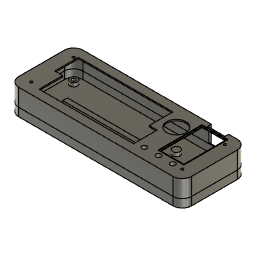
Macropad_V1_Case (Autodesk Fusion 360 design; units mm, degrees)
Autodesk Fusion 360 part; units mm, degrees
sketch "PCB" plane through (0, 0, 0) normal (0, 0, 1) x (1, 0, 0)
  line L0 (0, 0) -> (129.54, 0)
  line L1 (129.54, 0) -> (129.54, 41.91)
  line L2 (129.54, 41.91) -> (0, 41.91)
  line L3 (0, 41.91) -> (0, 0)
  circle A0 centre (3.81, 38.1) radius 1
  circle A1 centre (3.81, 3.81) radius 1
  circle A2 centre (125.73, 3.81) radius 1
  circle A3 centre (125.73, 38.1) radius 1
  line L4 (7.62, 38.1) -> (22.86, 38.1)
  line L5 (22.86, 38.1) -> (22.86, 22.86)
  line L6 (22.86, 22.86) -> (7.62, 22.86)
  line L7 (7.62, 22.86) -> (7.62, 38.1)
  line L8 (26.67, 22.86) -> (26.67, 38.1)
  line L9 (26.67, 38.1) -> (41.91, 38.1)
  line L10 (41.91, 38.1) -> (41.91, 22.86)
  line L11 (41.91, 22.86) -> (26.67, 22.86)
  line L12 (45.72, 22.86) -> (45.72, 38.1)
  line L13 (45.72, 38.1) -> (60.96, 38.1)
  line L14 (60.96, 38.1) -> (60.96, 22.86)
  line L15 (60.96, 22.86) -> (45.72, 22.86)
  line L16 (64.77, 22.86) -> (64.77, 38.1)
  line L17 (64.77, 38.1) -> (80.01, 38.1)
  line L18 (80.01, 38.1) -> (80.01, 22.86)
  line L19 (80.01, 22.86) -> (64.77, 22.86)
  line L20 (13.97, 19.05) -> (29.21, 19.05)
  line L21 (29.21, 19.05) -> (29.21, 3.81)
  line L22 (29.21, 3.81) -> (13.97, 3.81)
  line L23 (13.97, 3.81) -> (13.97, 19.05)
  line L24 (33.02, 3.81) -> (33.02, 19.05)
  line L25 (33.02, 19.05) -> (48.26, 19.05)
  line L26 (48.26, 19.05) -> (48.26, 3.81)
  line L27 (48.26, 3.81) -> (33.02, 3.81)
  line L28 (52.07, 3.81) -> (52.07, 19.05)
  line L29 (52.07, 19.05) -> (67.31, 19.05)
  line L30 (67.31, 19.05) -> (67.31, 3.81)
  line L31 (67.31, 3.81) -> (52.07, 3.81)
  line L32 (71.12, 3.81) -> (71.12, 19.05)
  line L33 (71.12, 19.05) -> (86.36, 19.05)
  line L34 (86.36, 19.05) -> (86.36, 3.81)
  line L35 (86.36, 3.81) -> (71.12, 3.81)
  line L36 (104.14, 41.91) -> (121.92, 41.91)
  line L37 (121.92, 41.91) -> (121.92, 8.89)
  line L38 (121.92, 8.89) -> (104.14, 8.89)
  line L39 (104.14, 8.89) -> (104.14, 41.91)
  line L40 (115.65, 6.27) -> (120.65, 6.27)
  line L41 (120.65, 6.27) -> (120.65, 1.27)
  line L42 (120.65, 1.27) -> (115.65, 1.27)
  line L43 (115.65, 1.27) -> (115.65, 6.27)
  line L44 (104.22, 1.27) -> (104.22, 6.27)
  line L45 (104.22, 6.27) -> (109.22, 6.27)
  line L46 (109.22, 6.27) -> (109.22, 1.27)
  line L47 (109.22, 1.27) -> (104.22, 1.27)
  line L48 (92.79, 1.27) -> (92.79, 6.27)
  line L49 (92.79, 6.27) -> (97.79, 6.27)
  line L50 (97.79, 6.27) -> (97.79, 1.27)
  line L51 (97.79, 1.27) -> (92.79, 1.27)
  circle A4 centre (93.98, 30.734) radius 3.81
  dimension "d1" = 129.54
  dimension "d2" = 41.91
  dimension "d38" = 2
  dimension "d39" = 3.81
  dimension "d40" = 3.81
  dimension "d41" = 2
  dimension "d42" = 3.81
  dimension "d43" = 3.81
  dimension "d44" = 2
  dimension "d45" = 3.81
  dimension "d46" = 3.81
  dimension "d47" = 2
  dimension "d48" = 3.81
  dimension "d49" = 3.81
  dimension "d50" = 15.24
  dimension "d51" = 15.24
  dimension "d52" = 7.62
  dimension "d53" = 3.81
  dimension "d56" = 19.05
  dimension "d57" = 0
  dimension "d58" = 15.24
  dimension "d59" = 15.24
  dimension "d60" = 19.05
  dimension "d61" = 6.35
  dimension "d64" = 19.05
  dimension "d65" = 0
  dimension "d66" = 17.78
  dimension "d67" = 33.02
  dimension "d68" = 7.62
  dimension "d71" = 5
  dimension "d72" = 5
  dimension "d73" = 8.89
  dimension "d74" = 1.27
  dimension "d77" = -11.43
  dimension "d78" = 0
  dimension "d79" = 7.62
  dimension "d80" = 35.56
  dimension "d81" = 11.176
  constraint horizontal L0
  constraint vertical L1
  constraint horizontal L2
  constraint vertical L3
  constraint coincident L0.start L3.end
  constraint horizontal L4
  constraint vertical L5
  constraint horizontal L6
  constraint vertical L7
  constraint horizontal L20
  constraint vertical L21
  constraint horizontal L22
  constraint vertical L23
  constraint horizontal L36
  constraint vertical L37
  constraint horizontal L38
  constraint vertical L39
  constraint collinear L2 L36
  constraint horizontal L40
  constraint vertical L41
  constraint horizontal L42
  constraint vertical L43
  measures "d1" distance of L0.start L0.end
  measures "d2" distance of L0.start L2.end
  measures "d38" diameter of A0
  measures "d39" distance of L3 A0.centre
  measures "d40" distance of L2 A0.centre
  measures "d41" diameter of A1
  measures "d42" distance of L0 A1.centre
  measures "d43" distance of L3 A1.centre
  measures "d44" diameter of A2
  measures "d45" distance of L1 A2.centre
  measures "d46" distance of L0 A2.centre
  measures "d47" diameter of A3
  measures "d48" distance of L2 A3.centre
  measures "d49" distance of L1 A3.centre
  measures "d50" distance of L4.start L4.end
  measures "d51" distance of L4.start L6.end
  measures "d52" distance of L3 L7
  measures "d53" distance of L2 L4
  measures "d58" distance of L20.end L20.start
  measures "d59" distance of L22.end L20.start
  measures "d60" distance of L4 L20
  measures "d61" distance of L7 L23
  measures "d66" distance of L36.start L36.end
  measures "d67" distance of L36.start L38.end
  measures "d68" distance of L1 L37
  measures "d71" distance of L40.start L40.end
  measures "d72" distance of L40.start L42.end
  measures "d73" distance of L1 L41
  measures "d74" distance of L0 L42
  measures "d79" diameter of A4
  measures "d80" distance of L1 A4.centre
  measures "d81" distance of L2 A4.centre
sketch "Bottom" plane through (0, 0, 0) normal (0, 0, 1) x (1, 0, 0)
  line L0 (2.5, 46.91) -> (127.04, 46.91)
  line L1 (134.54, 39.41) -> (134.54, 2.5)
  line L2 (127.04, -5) -> (2.5, -5)
  line L3 (-5, 2.5) -> (-5, 39.41)
  line L4 (0, 41.91) -> (0, 0)
  line L5 (129.54, 0) -> (129.54, 41.91)
  line L6 (129.54, 41.91) -> (0, 41.91)
  line L7 (0, 0) -> (129.54, 0)
  arc A0 (2.5, 46.91) -> (-5, 39.41) centre (2.5, 39.41) ccw
  arc A1 (134.54, 39.41) -> (127.04, 46.91) centre (127.04, 39.41) ccw
  arc A2 (127.04, -5) -> (134.54, 2.5) centre (127.04, 2.5) ccw
  arc A3 (-5, 2.5) -> (2.5, -5) centre (2.5, 2.5) ccw
  dimension "d9" = 5
  dimension "d10" = 5
  dimension "d11" = 5
  dimension "d12" = 5
  dimension "d13" = 7.5
  constraint horizontal L0
  constraint vertical L1
  constraint horizontal L2
  constraint vertical L3
  constraint tangent L3 A0
  constraint tangent L0 A0
  constraint tangent L0 A1
  constraint tangent L1 A1
  constraint equal A0 A1
  constraint tangent L1 A2
  constraint tangent L2 A2
  constraint equal A0 A2
  constraint tangent L2 A3
  constraint tangent L3 A3
  constraint equal A0 A3
  measures "d9" distance of L3 L4
  measures "d10" distance of L1 L5
  measures "d11" distance of L0 L6
  measures "d12" distance of L2 L7
  measures "d13" radius of A0
extrude "Extrude1" add sketch "Bottom" along normal blind 6.6 contours L0 L1 L2 L3 A0 A1 A2 A3 | L4 L5 L6 L7 makes body 1
sketch "Bottom indent" plane through (0, 0, 6.6) normal (0, 0, 1) x (-1, 0, 0)
  arc A0 (-2.5, -46.91) -> (5, -39.41) centre (-2.5, -39.41) ccw
  line L0 (5, -39.41) -> (5, -2.5)
  arc A1 (5, -2.5) -> (-2.5, 5) centre (-2.5, -2.5) ccw
  line L1 (-2.5, 5) -> (-127.04, 5)
  arc A2 (-127.04, 5) -> (-134.54, -2.5) centre (-127.04, -2.5) ccw
  line L2 (-134.54, -2.5) -> (-134.54, -39.41)
  arc A3 (-134.54, -39.41) -> (-127.04, -46.91) centre (-127.04, -39.41) ccw
  line L3 (-127.04, -46.91) -> (-2.5, -46.91)
  line L4 (-4.5, -44.91) -> (-125.04, -44.91)
  line L5 (-132.54, -37.41) -> (-132.54, -4.5)
  line L6 (-125.04, 3) -> (-4.5, 3)
  line L7 (3, -4.5) -> (3, -37.41)
  arc A4 (-4.5, -44.91) -> (3, -37.41) centre (-4.5, -37.41) ccw
  arc A5 (-132.54, -37.41) -> (-125.04, -44.91) centre (-125.04, -37.41) ccw
  arc A6 (-125.04, 3) -> (-132.54, -4.5) centre (-125.04, -4.5) ccw
  arc A7 (3, -4.5) -> (-4.5, 3) centre (-4.5, -4.5) ccw
  dimension "d17" = 2
  dimension "d18" = 2
  dimension "d19" = 2
  dimension "d20" = 2
  dimension "d21" = 7.5
  constraint horizontal L4
  constraint vertical L5
  constraint horizontal L6
  constraint vertical L7
  constraint tangent L7 A4
  constraint tangent L4 A4
  constraint tangent L4 A5
  constraint tangent L5 A5
  constraint equal A4 A5
  constraint tangent L5 A6
  constraint tangent L6 A6
  constraint equal A4 A6
  constraint tangent L6 A7
  constraint tangent L7 A7
  constraint equal A4 A7
  measures "d17" distance of L0 L7
  measures "d18" distance of L2 L5
  measures "d19" distance of L3 L4
  measures "d20" distance of L1 L6
  measures "d21" radius of A4
extrude "Extrude2" cut sketch "Bottom indent" against normal blind 4.6 contours L4 L5 L6 L7 A4 A5 A6 A7 bodies 1
sketch "Feet holes" plane through (0, 0, 0) normal (0, 0, -1) x (1, 0, 0)
  arc A0 (-5, -39.41) -> (2.5, -46.91) centre (2.5, -39.41) ccw
  line L0 (2.5, -46.91) -> (127.04, -46.91)
  arc A1 (127.04, -46.91) -> (134.54, -39.41) centre (127.04, -39.41) ccw
  line L1 (134.54, -39.41) -> (134.54, -2.5)
  arc A2 (134.54, -2.5) -> (127.04, 5) centre (127.04, -2.5) ccw
  line L2 (127.04, 5) -> (2.5, 5)
  arc A3 (2.5, 5) -> (-5, -2.5) centre (2.5, -2.5) ccw
  line L3 (-5, -2.5) -> (-5, -39.41)
  circle A4 centre (5, -5) radius 5
  circle A5 centre (5, -36.91) radius 5
  circle A6 centre (124.54, -5) radius 5
  circle A7 centre (124.54, -36.91) radius 5
  dimension "d24" = 10
  dimension "d25" = 10
  dimension "d26" = 10
  dimension "d27" = 10
  dimension "d28" = 10
  dimension "d29" = 10
  dimension "d30" = 10
  dimension "d31" = 10
  dimension "d32" = 10
  dimension "d33" = 10
  dimension "d34" = 10
  dimension "d35" = 10
  measures "d24" diameter of A4
  measures "d25" distance of L2 A4.centre
  measures "d26" distance of L3 A4.centre
  measures "d27" diameter of A5
  measures "d28" diameter of A6
  measures "d29" diameter of A7
  measures "d30" distance of L3 A5.centre
  measures "d31" distance of L0 A5.centre
  measures "d32" distance of L1 A6.centre
  measures "d33" distance of L2 A6.centre
  measures "d34" distance of L1 A7.centre
  measures "d35" distance of L0 A7.centre
extrude "Extrude3" cut sketch "Feet holes" against normal blind 1 contours A4 | A5 | A6 | A7 bodies 1
sketch "Bottom risers" plane through (0, 0, 2) normal (0, 0, 1) x (-1, 0, 0)
  arc A0 (-4.5, -44.91) -> (3, -37.41) centre (-4.5, -37.41) ccw
  line L0 (3, -37.41) -> (3, -4.5)
  arc A1 (3, -4.5) -> (-4.5, 3) centre (-4.5, -4.5) ccw
  line L1 (-4.5, 3) -> (-125.04, 3)
  arc A2 (-125.04, 3) -> (-132.54, -4.5) centre (-125.04, -4.5) ccw
  line L2 (-132.54, -4.5) -> (-132.54, -37.41)
  arc A3 (-132.54, -37.41) -> (-125.04, -44.91) centre (-125.04, -37.41) ccw
  line L3 (-125.04, -44.91) -> (-4.5, -44.91)
  circle A4 centre (-3.81, -38.1) radius 3
  circle A5 centre (-3.81, -38.1) radius 1
  circle A6 centre (-3.81, -3.81) radius 3
  circle A7 centre (-125.73, -38.1) radius 3
  circle A8 centre (-125.73, -3.81) radius 3
  circle A9 centre (-3.81, -3.81) radius 1
  circle A10 centre (-125.73, -38.1) radius 1
  circle A11 centre (-125.73, -3.81) radius 1
  line L4 (-13.97, -22.86) -> (-80.01, -22.86)
  line L5 (-80.01, -22.86) -> (-80.01, -19.05)
  line L6 (-80.01, -19.05) -> (-13.97, -19.05)
  line L7 (-13.97, -19.05) -> (-13.97, -22.86)
  line L8 (-80.01, -38.1) -> (-80.01, -22.86)
  line L9 (-13.97, -3.81) -> (-13.97, -19.05)
  line L10 (-13.97, -19.05) -> (-29.21, -19.05)
  line L11 (-80.01, -22.86) -> (-64.77, -22.86)
  circle A12 centre (-93.98, -30.734) radius 3
  circle A13 centre (-93.98, -30.734) radius 3.81
  circle A14 centre (-3.81, -38.1) radius 1.5
  circle A15 centre (-3.81, -3.81) radius 1.5
  circle A16 centre (-125.73, -3.81) radius 1.5
  circle A17 centre (-125.73, -38.1) radius 1.5
  dimension "d82" = 6
  dimension "d83" = 6
  dimension "d84" = 6
  dimension "d85" = 6
  dimension "d87" = 6
  dimension "d88" = 3
  dimension "d89" = 3
  dimension "d90" = 3
  dimension "d91" = 3
  constraint concentric A4 A5
  constraint concentric A6 A9
  constraint concentric A7 A10
  constraint concentric A8 A11
  constraint horizontal L4
  constraint vertical L5
  constraint horizontal L6
  constraint vertical L7
  constraint collinear L5 L8
  constraint collinear L7 L9
  constraint collinear L6 L10
  constraint collinear L4 L11
  constraint concentric A12 A13
  constraint concentric A5 A14
  constraint concentric A9 A15
  constraint concentric A11 A16
  constraint concentric A10 A17
  measures "d82" diameter of A4
  measures "d83" diameter of A6
  measures "d84" diameter of A7
  measures "d85" diameter of A8
  measures "d87" diameter of A12
  measures "d88" diameter of A14
  measures "d89" diameter of A15
  measures "d90" diameter of A16
  measures "d91" diameter of A17
extrude "Extrude4" add sketch "Bottom risers" along normal blind 3 contours A4 | A6 | A7 | A8 | L4 L5 L6 L7 L10 L11 | A12 bodies 1
extrude "Extrude5" cut 4 faces at (4.4705, 37.7379, 2) (3.6858, 4.5903, 2) (125.6187, 38.5875, 2) (126.2643, 4.2009, 2) along direction (0, 0, -1) blind 1 on bodies 1 bodies 1
sketch "Bottom Raised Edge" plane through (0, 0, 6.6) normal (0, 0, 1) x (-1, 0, 0)
  line L0 (3, -4.5) -> (3, -37.41)
  arc A0 (-4.5, -44.91) -> (3, -37.41) centre (-4.5, -37.41) ccw
  line L1 (-4.5, -44.91) -> (-125.04, -44.91)
  arc A1 (-132.54, -37.41) -> (-125.04, -44.91) centre (-125.04, -37.41) ccw
  line L2 (-132.54, -37.41) -> (-132.54, -4.5)
  arc A2 (-125.04, 3) -> (-132.54, -4.5) centre (-125.04, -4.5) ccw
  line L3 (-125.04, 3) -> (-4.5, 3)
  arc A3 (3, -4.5) -> (-4.5, 3) centre (-4.5, -4.5) ccw
  arc A4 (-2.5, -46.91) -> (5, -39.41) centre (-2.5, -39.41) ccw
  line L4 (5, -39.41) -> (5, -2.5)
  arc A5 (5, -2.5) -> (-2.5, 5) centre (-2.5, -2.5) ccw
  line L5 (-2.5, 5) -> (-127.04, 5)
  arc A6 (-127.04, 5) -> (-134.54, -2.5) centre (-127.04, -2.5) ccw
  line L6 (-134.54, -2.5) -> (-134.54, -39.41)
  arc A7 (-134.54, -39.41) -> (-127.04, -46.91) centre (-127.04, -39.41) ccw
  line L7 (-127.04, -46.91) -> (-2.5, -46.91)
  line L8 (-3.7, -45.71) -> (-125.84, -45.71)
  line L9 (-133.34, -38.21) -> (-133.34, -3.7)
  line L10 (-125.84, 3.8) -> (-3.7, 3.8)
  line L11 (3.8, -3.7) -> (3.8, -38.21)
  arc A8 (-3.7, -45.71) -> (3.8, -38.21) centre (-3.7, -38.21) ccw
  arc A9 (-133.34, -38.21) -> (-125.84, -45.71) centre (-125.84, -38.21) ccw
  arc A10 (-125.84, 3.8) -> (-133.34, -3.7) centre (-125.84, -3.7) ccw
  arc A11 (3.8, -3.7) -> (-3.7, 3.8) centre (-3.7, -3.7) ccw
  dimension "d96" = 0.8
  dimension "d97" = 0.8
  dimension "d98" = 0.8
  dimension "d100" = 0.8
  dimension "d101" = 7.5
  constraint horizontal L8
  constraint vertical L9
  constraint horizontal L10
  constraint vertical L11
  constraint tangent L8 A8
  constraint tangent L11 A8
  constraint tangent L8 A9
  constraint tangent L9 A9
  constraint equal A8 A9
  constraint tangent L9 A10
  constraint tangent L10 A10
  constraint equal A8 A10
  constraint tangent L10 A11
  constraint tangent L11 A11
  constraint equal A8 A11
  measures "d96" distance of L1 L8
  measures "d97" distance of L0 L11
  measures "d98" distance of L2 L9
  measures "d100" distance of L3 L10
  measures "d101" radius of A8
extrude "Extrude6" add sketch "Bottom Raised Edge" along normal blind 1.4 contours L8 L9 L10 L11 A8 A9 A10 A11 bodies 1
sketch "Top" plane through (0, 0, 6.6) normal (0, 0, 1) x (-1, 0, 0)
  line L0 (-3.7, -45.71) -> (-125.84, -45.71)
  arc A0 (-133.34, -38.21) -> (-125.84, -45.71) centre (-125.84, -38.21) ccw
  line L1 (-133.34, -38.21) -> (-133.34, -3.7)
  arc A1 (-125.84, 3.8) -> (-133.34, -3.7) centre (-125.84, -3.7) ccw
  line L2 (-125.84, 3.8) -> (-3.7, 3.8)
  arc A2 (3.8, -3.7) -> (-3.7, 3.8) centre (-3.7, -3.7) ccw
  line L3 (3.8, -3.7) -> (3.8, -38.21)
  arc A3 (-3.7, -45.71) -> (3.8, -38.21) centre (-3.7, -38.21) ccw
  arc A4 (-2.5, -46.91) -> (5, -39.41) centre (-2.5, -39.41) ccw
  line L4 (5, -39.41) -> (5, -2.5)
  arc A5 (5, -2.5) -> (-2.5, 5) centre (-2.5, -2.5) ccw
  line L5 (-2.5, 5) -> (-127.04, 5)
  arc A6 (-127.04, 5) -> (-134.54, -2.5) centre (-127.04, -2.5) ccw
  line L6 (-134.54, -2.5) -> (-134.54, -39.41)
  arc A7 (-134.54, -39.41) -> (-127.04, -46.91) centre (-127.04, -39.41) ccw
  line L7 (-127.04, -46.91) -> (-2.5, -46.91)
  line L8 (-2.5, -46.91) -> (-127.04, -46.91)
  line L9 (-134.54, -39.41) -> (-134.54, -2.5)
  line L10 (-127.04, 5) -> (-2.5, 5)
  line L11 (5, -2.5) -> (5, -39.41)
  arc A8 (-2.5, -46.91) -> (5, -39.41) centre (-2.5, -39.41) ccw
  arc A9 (-134.54, -39.41) -> (-127.04, -46.91) centre (-127.04, -39.41) ccw
  arc A10 (-127.04, 5) -> (-134.54, -2.5) centre (-127.04, -2.5) ccw
  arc A11 (5, -2.5) -> (-2.5, 5) centre (-2.5, -2.5) ccw
  dimension "d105" = 7.5
  constraint horizontal L8
  constraint vertical L9
  constraint horizontal L10
  constraint vertical L11
  constraint collinear L7 L8
  constraint collinear L4 L11
  constraint collinear L5 L10
  constraint collinear L6 L9
  constraint tangent L8 A8
  constraint tangent L11 A8
  constraint tangent L8 A9
  constraint tangent L9 A9
  constraint equal A8 A9
  constraint tangent L9 A10
  constraint tangent L10 A10
  constraint equal A8 A10
  constraint tangent L10 A11
  constraint tangent L11 A11
  constraint equal A8 A11
  measures "d105" radius of A8
extrude "Extrude7" add sketch "Top" along normal blind 14 separate body contours L0 A0 L1 A1 L2 A2 L3 A3 | A4 L4 A5 L5 A6 L6 A7 L7 L8 L9 L10 L11 A8 A9 A10 A11 makes body 2
sketch "Top Indent" plane through (0, 0, 6.6) normal (0, 0, -1) x (1, 0, 0)
  arc A0 (-5, -39.41) -> (2.5, -46.91) centre (2.5, -39.41) ccw
  line L0 (2.5, -46.91) -> (127.04, -46.91)
  arc A1 (127.04, -46.91) -> (134.54, -39.41) centre (127.04, -39.41) ccw
  line L1 (134.54, -39.41) -> (134.54, -2.5)
  arc A2 (134.54, -2.5) -> (127.04, 5) centre (127.04, -2.5) ccw
  line L2 (127.04, 5) -> (2.5, 5)
  arc A3 (2.5, 5) -> (-5, -2.5) centre (2.5, -2.5) ccw
  line L3 (-5, -2.5) -> (-5, -39.41)
  line L4 (4.5, 3) -> (125.04, 3)
  line L5 (132.54, -4.5) -> (132.54, -37.41)
  line L6 (125.04, -44.91) -> (4.5, -44.91)
  line L7 (-3, -37.41) -> (-3, -4.5)
  arc A4 (4.5, 3) -> (-3, -4.5) centre (4.5, -4.5) ccw
  arc A5 (132.54, -4.5) -> (125.04, 3) centre (125.04, -4.5) ccw
  arc A6 (125.04, -44.91) -> (132.54, -37.41) centre (125.04, -37.41) ccw
  arc A7 (-3, -37.41) -> (4.5, -44.91) centre (4.5, -37.41) ccw
  dimension "d109" = 2
  dimension "d110" = 2
  dimension "d111" = 2
  dimension "d112" = 2
  dimension "d113" = 7.5
  constraint horizontal L4
  constraint vertical L5
  constraint horizontal L6
  constraint vertical L7
  constraint tangent L4 A4
  constraint tangent L7 A4
  constraint tangent L4 A5
  constraint tangent L5 A5
  constraint equal A4 A5
  constraint tangent L5 A6
  constraint tangent L6 A6
  constraint equal A4 A6
  constraint tangent L6 A7
  constraint tangent L7 A7
  constraint equal A4 A7
  measures "d109" distance of L2 L4
  measures "d110" distance of L0 L6
  measures "d111" distance of L3 L7
  measures "d112" distance of L1 L5
  measures "d113" radius of A4
extrude "Extrude8" cut sketch "Top Indent" against normal blind 13 contours L4 L5 L6 L7 A4 A5 A6 A7 bodies 2
sketch "Top Light Pipes" plane through (0, 0, 19.6) normal (0, 0, -1) x (1, 0, 0)
  arc A0 (4.5, 3) -> (-3, -4.5) centre (4.5, -4.5) ccw
  line L0 (-3, -4.5) -> (-3, -37.41)
  arc A1 (-3, -37.41) -> (4.5, -44.91) centre (4.5, -37.41) ccw
  line L1 (4.5, -44.91) -> (125.04, -44.91)
  arc A2 (125.04, -44.91) -> (132.54, -37.41) centre (125.04, -37.41) ccw
  line L2 (132.54, -37.41) -> (132.54, -4.5)
  arc A3 (132.54, -4.5) -> (125.04, 3) centre (125.04, -4.5) ccw
  line L3 (125.04, 3) -> (4.5, 3)
  circle A4 centre (118.15, -3.77) radius 3
  circle A5 centre (-95.29, -3.77) radius 2
  circle A6 centre (106.72, -3.77) radius 3
  circle A7 centre (95.29, -3.77) radius 3
  line L4 (115.65, -6.27) -> (120.65, -6.27)
  line L5 (115.65, -1.27) -> (115.65, -6.27)
  line L6 (104.22, -6.27) -> (109.22, -6.27)
  line L7 (104.22, -1.27) -> (104.22, -6.27)
  line L8 (92.79, -6.27) -> (97.79, -6.27)
  line L9 (92.79, -1.27) -> (92.79, -6.27)
  dimension "d168" = 6
  dimension "d169" = 4
  dimension "d170" = 6
  dimension "d171" = 6
  dimension "d172" = 2.5
  dimension "d173" = 2.5
  dimension "d174" = 2.5
  dimension "d175" = 2.5
  dimension "d176" = 2.5
  dimension "d177" = 2.5
  measures "d168" diameter of A4
  measures "d169" diameter of A5
  measures "d170" diameter of A6
  measures "d171" diameter of A7
  measures "d172" distance of A4.centre L4
  measures "d173" distance of A4.centre L5
  measures "d174" distance of A6.centre L6
  measures "d175" distance of A6.centre L7
  measures "d176" distance of A7.centre L8
  measures "d177" distance of A7.centre L9
extrude "Extrude12" add sketch "Top Light Pipes" along normal blind 11 contours A4 L4 L5 | A4 L5 | A4 L4 | A6 L6 L7 | A6 L7 | A6 L6 | A7 L8 L9 | A7 L9 | A7 L8 picked at (118.1589, -4.4367) picked at (106.7289, -4.4367) picked at (95.2989, -4.4367) bodies 2
sketch "Top Key Holes" plane through (0, 0, 20.6) normal (0, 0, 1) x (-1, 0, 0)
  arc A0 (-2.5, -46.91) -> (5, -39.41) centre (-2.5, -39.41) ccw
  line L0 (5, -39.41) -> (5, -2.5)
  arc A1 (5, -2.5) -> (-2.5, 5) centre (-2.5, -2.5) ccw
  line L1 (-2.5, 5) -> (-127.04, 5)
  arc A2 (-127.04, 5) -> (-134.54, -2.5) centre (-127.04, -2.5) ccw
  line L2 (-134.54, -2.5) -> (-134.54, -39.41)
  arc A3 (-134.54, -39.41) -> (-127.04, -46.91) centre (-127.04, -39.41) ccw
  line L3 (-127.04, -46.91) -> (-2.5, -46.91)
  line L4 (-5.715, -40.005) -> (-24.765, -40.005)
  line L5 (-24.765, -40.005) -> (-24.765, -20.955)
  line L6 (-24.765, -20.955) -> (-5.715, -20.955)
  line L7 (-5.715, -20.955) -> (-5.715, -40.005)
  line L8 (-7.62, -38.1) -> (-22.86, -38.1)
  line L9 (-7.62, -22.86) -> (-7.62, -38.1)
  line L10 (-43.815, -20.955) -> (-24.765, -20.955)
  line L11 (-24.765, -20.955) -> (-24.765, -40.005)
  line L12 (-24.765, -40.005) -> (-43.815, -40.005)
  line L13 (-43.815, -40.005) -> (-43.815, -20.955)
  line L14 (-62.865, -20.955) -> (-43.815, -20.955)
  line L15 (-43.815, -20.955) -> (-43.815, -40.005)
  line L16 (-43.815, -40.005) -> (-62.865, -40.005)
  line L17 (-62.865, -40.005) -> (-62.865, -20.955)
  line L18 (-81.915, -20.955) -> (-62.865, -20.955)
  line L19 (-62.865, -20.955) -> (-62.865, -40.005)
  line L20 (-62.865, -40.005) -> (-81.915, -40.005)
  line L21 (-81.915, -40.005) -> (-81.915, -20.955)
  line L22 (-31.115, -1.905) -> (-12.065, -1.905)
  line L23 (-12.065, -1.905) -> (-12.065, -20.955)
  line L24 (-12.065, -20.955) -> (-31.115, -20.955)
  line L25 (-31.115, -20.955) -> (-31.115, -1.905)
  line L26 (-13.97, -3.81) -> (-13.97, -19.05)
  line L27 (-29.21, -3.81) -> (-13.97, -3.81)
  line L28 (-50.165, -20.955) -> (-50.165, -1.905)
  line L29 (-50.165, -1.905) -> (-31.115, -1.905)
  line L30 (-31.115, -1.905) -> (-31.115, -20.955)
  line L31 (-31.115, -20.955) -> (-50.165, -20.955)
  line L32 (-69.215, -20.955) -> (-69.215, -1.905)
  line L33 (-69.215, -1.905) -> (-50.165, -1.905)
  line L34 (-50.165, -1.905) -> (-50.165, -20.955)
  line L35 (-50.165, -20.955) -> (-69.215, -20.955)
  line L36 (-88.265, -20.955) -> (-88.265, -1.905)
  line L37 (-88.265, -1.905) -> (-69.215, -1.905)
  line L38 (-69.215, -1.905) -> (-69.215, -20.955)
  line L39 (-69.215, -20.955) -> (-88.265, -20.955)
  circle A4 centre (-93.98, -30.734) radius 7.75
  line L40 (-103.64, -42.41) -> (-122.42, -42.41)
  line L41 (-122.42, -42.41) -> (-122.42, -8.39)
  line L42 (-122.42, -8.39) -> (-103.64, -8.39)
  line L43 (-103.64, -8.39) -> (-103.64, -42.41)
  line L44 (-121.92, -41.91) -> (-121.92, -8.89)
  line L45 (-104.14, -8.89) -> (-104.14, -41.91)
  line L46 (-129.54, -41.91) -> (0, -41.91)
  line L47 (-121.92, -8.89) -> (-104.14, -8.89)
  circle A5 centre (-125.73, -38.1) radius 1
  circle A6 centre (-125.73, -3.81) radius 1
  circle A7 centre (-3.81, -38.1) radius 1
  circle A8 centre (-3.81, -3.81) radius 1
  circle A9 centre (-95.29, -3.77) radius 2
  circle A10 centre (-106.72, -3.77) radius 2
  circle A11 centre (-118.15, -3.77) radius 2
  circle A12 centre (-95.29, -3.77) radius 3
  circle A13 centre (-106.72, -3.77) radius 3
  circle A14 centre (-118.15, -3.77) radius 3
  line L48 (-106.03, -46.91) -> (-120.03, -46.91)
  line L49 (-120.03, -46.91) -> (-120.03, -43.91)
  line L50 (-120.03, -43.91) -> (-106.03, -43.91)
  line L51 (-106.03, -43.91) -> (-106.03, -46.91)
  point P0 (-93.98, -30.734)
  point P1 (-3.81, -3.81)
  point P2 (-3.81, -38.1)
  point P3 (-125.73, -38.1)
  point P4 (-125.73, -3.81)
  dimension "d116" = 19.05
  dimension "d117" = 19.05
  dimension "d118" = 1.905
  dimension "d119" = 1.905
  dimension "d122" = -19.05
  dimension "d123" = 0
  dimension "d124" = 19.05
  dimension "d125" = 19.05
  dimension "d126" = 1.905
  dimension "d127" = 1.905
  dimension "d130" = -19.05
  dimension "d131" = 0
  dimension "d132" = 15.5
  dimension "d134" = 0.5
  dimension "d135" = 0.5
  dimension "d136" = 0.5
  dimension "d137" = 0.5
  dimension "d138" = 2
  dimension "d139" = 2
  dimension "d140" = 2
  dimension "d141" = 2
  dimension "d159" = 4
  dimension "d160" = 4
  dimension "d161" = 4
  dimension "d183" = 14
  dimension "d184" = 2
  dimension "d186" = 1.89
  constraint horizontal L4
  constraint vertical L5
  constraint horizontal L6
  constraint vertical L7
  constraint horizontal L24
  constraint vertical L25
  constraint horizontal L22
  constraint vertical L23
  constraint coincident P0 A4.centre
  constraint horizontal L40
  constraint vertical L41
  constraint horizontal L42
  constraint vertical L43
  constraint coincident P1 A8.centre
  constraint coincident P2 A7.centre
  constraint coincident P3 A5.centre
  constraint coincident P4 A6.centre
  constraint concentric A9 A12
  constraint concentric A10 A13
  constraint concentric A11 A14
  constraint horizontal L48
  constraint vertical L49
  constraint horizontal L50
  constraint vertical L51
  constraint collinear L3 L48
  measures "d116" distance of L4.start L4.end
  measures "d117" distance of L4.start L6.end
  measures "d118" distance of L4 L8
  measures "d119" distance of L7 L9
  measures "d124" distance of L23.end L24.end
  measures "d125" distance of L22.end L23.end
  measures "d126" distance of L23 L26
  measures "d127" distance of L22 L27
  measures "d132" diameter of A4
  measures "d134" distance of L41 L44
  measures "d135" distance of L43 L45
  measures "d136" distance of L40 L46
  measures "d137" distance of L42 L47
  measures "d138" diameter of A5
  measures "d139" diameter of A6
  measures "d140" diameter of A7
  measures "d141" diameter of A8
  measures "d159" diameter of A9
  measures "d160" diameter of A10
  measures "d161" diameter of A11
  measures "d183" distance of L48.start L48.end
  measures "d184" distance of L46 L50
  measures "d186" distance of L45 L51
extrude "Extrude9" cut sketch "Top Key Holes" against normal blind 14 contours L3 L48 L49 L50 L51 | L4 L5 L6 L7 L11 L24 | L5 L10 L11 L12 L13 L15 L24 L31 | L6 L10 L22 L23 L24 L25 L30 | L13 L14 L15 L16 L17 L19 L31 L35 | L10 L14 L25 L28 L29 L30 L31 L34 | L17 L18 L19 L20 L21 L35 L39 | L14 L18 L28 L32 L33 L34 L35 L38 | L18 L32 L36 L37 L38 L39 | A4 | L41 L42 L43 L44 L45 L46 L47 | L44 L45 L46 L47 | A5 | A6 | A7 | A8 | A9 | A10 | A11 bodies 2
sketch "Top Raised Edge" plane through (0, 0, 6.6) normal (0, 0, -1) x (1, 0, 0)
  line L0 (-3, -37.41) -> (-3, -4.5)
  arc A0 (4.5, 3) -> (-3, -4.5) centre (4.5, -4.5) ccw
  line L1 (4.5, 3) -> (125.04, 3)
  arc A1 (132.54, -4.5) -> (125.04, 3) centre (125.04, -4.5) ccw
  line L2 (132.54, -4.5) -> (132.54, -37.41)
  arc A2 (125.04, -44.91) -> (132.54, -37.41) centre (125.04, -37.41) ccw
  line L3 (106.03, -44.91) -> (4.5, -44.91)
  arc A3 (-3, -37.41) -> (4.5, -44.91) centre (4.5, -37.41) ccw
  arc A4 (-5, -39.41) -> (2.5, -46.91) centre (2.5, -39.41) ccw
  line L4 (120.03, -46.91) -> (127.04, -46.91)
  arc A5 (127.04, -46.91) -> (134.54, -39.41) centre (127.04, -39.41) ccw
  line L5 (134.54, -39.41) -> (134.54, -2.5)
  arc A6 (134.54, -2.5) -> (127.04, 5) centre (127.04, -2.5) ccw
  line L6 (127.04, 5) -> (2.5, 5)
  arc A7 (2.5, 5) -> (-5, -2.5) centre (2.5, -2.5) ccw
  line L7 (-5, -2.5) -> (-5, -39.41)
  line L8 (3.3, 4.2) -> (126.24, 4.2)
  line L9 (133.74, -3.3) -> (133.74, -38.61)
  line L10 (126.24, -46.11) -> (3.3, -46.11)
  line L11 (-4.2, -38.61) -> (-4.2, -3.3)
  arc A8 (3.3, 4.2) -> (-4.2, -3.3) centre (3.3, -3.3) ccw
  arc A9 (133.74, -3.3) -> (126.24, 4.2) centre (126.24, -3.3) ccw
  arc A10 (126.24, -46.11) -> (133.74, -38.61) centre (126.24, -38.61) ccw
  arc A11 (-4.2, -38.61) -> (3.3, -46.11) centre (3.3, -38.61) ccw
  line L12 (120.03, -44.91) -> (120.03, -46.91)
  line L13 (2.5, -46.91) -> (106.03, -46.91)
  line L14 (106.03, -46.91) -> (106.03, -44.91)
  line L15 (125.04, -44.91) -> (120.03, -44.91)
  dimension "d145" = 0.8
  dimension "d146" = 0.8
  dimension "d147" = 0.8
  dimension "d148" = 0.8
  dimension "d149" = 7.5
  constraint horizontal L8
  constraint vertical L9
  constraint horizontal L10
  constraint vertical L11
  constraint tangent L8 A8
  constraint tangent L11 A8
  constraint tangent L8 A9
  constraint tangent L9 A9
  constraint equal A8 A9
  constraint tangent L9 A10
  constraint tangent L10 A10
  constraint equal A8 A10
  constraint tangent L10 A11
  constraint tangent L11 A11
  constraint equal A8 A11
  measures "d145" distance of L6 L8
  measures "d146" distance of L7 L11
  measures "d147" distance of L4 L10
  measures "d148" distance of L5 L9
  measures "d149" radius of A8
extrude "Extrude10" cut sketch "Top Raised Edge" against normal blind 1.4 contours L0 A0 L1 A1 L2 A2 L3 A3 L8 L9 L10 L11 A8 A9 A10 A11 L12 L14 L15 bodies 2
sketch "Top Window Indent" plane through (0, 0, 20.6) normal (0, 0, 1) x (-1, 0, 0)
  circle A0 centre (-3.81, -3.81) radius 1
  line L0 (-5.715, -20.955) -> (-5.715, -40.005)
  line L1 (-5.715, -40.005) -> (-81.915, -40.005)
  line L2 (-81.915, -40.005) -> (-81.915, -20.955)
  line L3 (-81.915, -20.955) -> (-88.265, -20.955)
  line L4 (-88.265, -20.955) -> (-88.265, -1.905)
  line L5 (-88.265, -1.905) -> (-12.065, -1.905)
  line L6 (-12.065, -1.905) -> (-12.065, -20.955)
  line L7 (-12.065, -20.955) -> (-5.715, -20.955)
  circle A1 centre (-125.73, -3.81) radius 1
  circle A2 centre (-3.81, -38.1) radius 1
  circle A3 centre (-93.98, -30.734) radius 7.75
  line L8 (-103.64, -8.39) -> (-103.64, -41.91)
  line L9 (-103.64, -41.91) -> (-122.42, -41.91)
  line L10 (-122.42, -41.91) -> (-122.42, -8.39)
  line L11 (-122.42, -8.39) -> (-103.64, -8.39)
  circle A4 centre (-125.73, -38.1) radius 1
  arc A5 (-2.5, -46.91) -> (5, -39.41) centre (-2.5, -39.41) ccw
  line L12 (5, -39.41) -> (5, -2.5)
  arc A6 (5, -2.5) -> (-2.5, 5) centre (-2.5, -2.5) ccw
  line L13 (-2.5, 5) -> (-127.04, 5)
  arc A7 (-127.04, 5) -> (-134.54, -2.5) centre (-127.04, -2.5) ccw
  line L14 (-134.54, -2.5) -> (-134.54, -39.41)
  arc A8 (-134.54, -39.41) -> (-127.04, -46.91) centre (-127.04, -39.41) ccw
  line L15 (-106.03, -46.91) -> (-2.5, -46.91)
  line L16 (-102.64, -42.91) -> (-123.42, -42.91)
  line L17 (-123.42, -42.91) -> (-123.42, -7.39)
  line L18 (-123.42, -7.39) -> (-102.64, -7.39)
  line L19 (-102.64, -7.39) -> (-102.64, -42.91)
  circle A9 centre (-95.29, -3.77) radius 2
  circle A10 centre (-106.72, -3.77) radius 2
  circle A11 centre (-118.15, -3.77) radius 2
  line L20 (-120.03, -46.91) -> (-120.03, -43.91)
  line L21 (-120.03, -43.91) -> (-106.03, -43.91)
  line L22 (-106.03, -43.91) -> (-106.03, -46.91)
  line L23 (-127.04, -46.91) -> (-120.03, -46.91)
  dimension "d153" = 1
  dimension "d154" = 1
  dimension "d155" = 1
  dimension "d156" = 1
  constraint horizontal L16
  constraint vertical L17
  constraint horizontal L18
  constraint vertical L19
  measures "d153" distance of L9 L16
  measures "d154" distance of L10 L17
  measures "d155" distance of L11 L18
  measures "d156" distance of L8 L19
extrude "Extrude11" cut sketch "Top Window Indent" against normal blind 0.5 contours L16 L17 L18 L19 bodies 2
equation "d14 = 2 mm + 3 mm + 1.6 mm"
equation "d22 = -3 mm - 1.6 mm"
equation "d77 = ( -4.5 * 2.54 ) * 1 mm"
equation "d118 = ( ( 19.05 - 15.24 ) / 2 ) * 1 mm"
equation "d119 = ( ( 19.05 - 15.24 ) / 2 ) * 1 mm"
equation "d126 = ( ( 19.05 - 15.24 ) / 2 ) * 1 mm"
equation "d127 = ( ( 19.05 - 15.24 ) / 2 ) * 1 mm"
equation "d178 = 14 mm - 1 mm - 2 mm"
equation "d186 = ( ( 17.78 - 14 ) / 2 ) * 1 mm"
named bodies: "Bottom", "Top"
